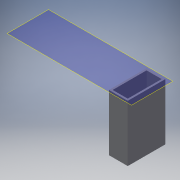
# Autodesk Inventor part: bar thing
Saved by Autodesk Inventor 2018 (Build 220112000, 112)
## iProperties
Created: 2019-01-26
Part Number: bar thing
Material: Generic
Document SubType Name: Modeling
Designer: s-4008082
Density: 1 g/cm^3
Appearance: Default
Author: s-4008082
Autodesk Inventor part; units mm, degrees
ref_plane "YZ Plane" through (0, 0, 0) normal (1, 0, 0) x (0, 1, 0)
ref_plane "XZ Plane" through (0, 0, 0) normal (0, 1, 0) x (-1, 0, 0)
ref_plane "XY Plane" through (0, 0, 0) normal (0, 0, 1) x (1, 0, 0)
ref_plane "Work Plane1" through (50.8, -12.7, 0) normal (0, -1, 0) x (0, 0, 1)
sketch "Sketch1" plane through (50.8, -12.7, 0) normal (0, -1, 0) x (0, 0, 1)
  line L0 (-0.1298, 0) -> (50.6702, 0)
  line L1 (50.6702, 0) -> (50.6702, 25.4)
  line L2 (50.6702, 25.4) -> (-0.1298, 25.4)
  line L3 (-0.1298, 25.4) -> (-0.1298, 0)
  line L4 (48.1302, 22.86) -> (2.4102, 22.86)
  line L5 (2.4102, 22.86) -> (2.4102, 2.54)
  line L6 (2.4102, 2.54) -> (48.1302, 2.54)
  line L7 (48.1302, 2.54) -> (48.1302, 22.86)
  point P0 (0, 50.8)
  dimension "d0" = 25.4
  dimension "d1" = 50.8
  dimension "d3" = 2.54
  dimension "d4" = 2.54
  dimension "d5" = 2.54
  dimension "d6" = 2.54
  constraints: 16 end point, 4 parallel, 2 horizontal, 2 perpendicular
  measures "d0" distance of L0.end L1.end
  measures "d1" distance of L1.end L2.end
  measures "d3" distance between parallel lines of L3 L5
  measures "d4" distance between parallel lines of L0 L6
  measures "d5" distance between parallel lines of L2 L4
  measures "d6" distance between parallel lines of L1 L7
extrude "Extrusion1" add sketch "Sketch1" along normal blind 76.2
sketch "Sketch2" plane through (25.4, -12.7, 50.6702) normal (0, 0, 1) x (1, 0, 0)
  circle A0 centre (12.7, -12.7) radius 2.5797
  circle A1 centre (12.7, -38.1) radius 2.5797
  line L0 (25.4, 0) -> (0, 0) projected
  line L1 (0, 0) -> (0, -76.2) projected
  point P0 (-25.4, 12.7)
  dimension "d9" = 12.7
  dimension "d10" = 25.4
  dimension "d11" = 5.1594
  dimension "d12" = 5.1594
  dimension "d13" = 12.7
  dimension "d14" = 12.7
  constraints: 2 centre point
  measures "d9" distance from line of L0 A0.centre
  measures "d10" distance of A0.centre A1.centre
  measures "d11" diameter of A1
  measures "d12" diameter of A0
  measures "d13" distance from line of L1 A0.centre
  measures "d14" distance from line of L1 A1.centre
extrude "Extrusion2" cut sketch "Sketch2" against normal blind 76.2
body "Solid1"
